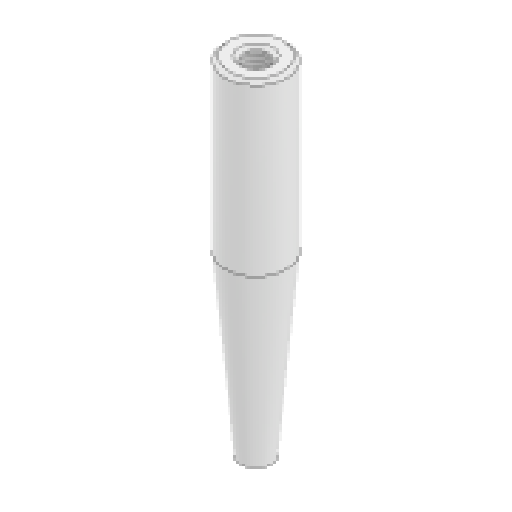
# Autodesk Inventor part: DLT-01-238B
Saved by Autodesk Inventor 2025.2 (Build 292293000, 293)
## iProperties
Company: Delta
Created: 2024-10-22
Part Number: DLT-01-238B
Material: Poliacetal WT
Document SubType Name: Modeling
Designer: Willian Pinheiro
Density: 1.4 g/cm^3
Appearance: Smooth - White
Project: DLT-01
Description: Dedo Pressor B
Mass: 13.0552 g
Surface Area: 40.3439 cm^2
Volume: 9.32516 cm^3
Acabamento: N/A
Dimensões: Ø10 x 45 mm
Total: 1
Author: Willian Pinheiro
Revision Number: 00
Autodesk Inventor part; units mm, degrees
ref_plane "YZ Plane" through (0, 0, 0) normal (1, 0, 0) x (0, 1, 0)
ref_plane "XZ Plane" through (0, 0, 0) normal (0, 1, 0) x (-1, 0, 0)
ref_plane "XY Plane" through (0, 0, 0) normal (0, 0, 1) x (1, 0, 0)
sketch "Sketch1" plane through (0, 0, 0) normal (0, 1, 0) x (-1, 0, 0)
  line L0 (4.8, 0) -> (-0.8, 0) construction
  line L1 (0, -37.7337) -> (0, 68.9023) construction
  line L2 (4, 22.5) -> (0, 22.5)
  line L3 (0, 22.5) -> (0, -22.5)
  line L4 (0, -22.5) -> (4, -22.5)
  line L5 (4, -22.5) -> (4, 22.5)
  line L6 (4, 53.6686) -> (4, 38.3314)
  line L7 (1.9878, -22.5) -> (4, 0.5)
  point P0 (0, 0)
  point P1 (0, 22.5)
  point P2 (0, -22.5)
  dimension "d2" = 8
  dimension "d5" = 23
  dimension "d21" = 45
  dimension "d22" = 3.9755
  dimension "d23" = 5
  constraints: 12 end point, 2 collinear, 2 parallel, 2 point on line, 1 horizontal, 1 perpendicular, 1 other
  measures "d2" diameter of L5 L1
  measures "d5" vertical distance of L7.start L7.end
  measures "d21" distance between parallel lines of L4 L2
  measures "d22" diameter of L7.start L1
  measures "d23" angle of L5 L7
revolve "Revolution1" add sketch "Sketch1" angle 360 about axis through (0, 0, -10) along (0, 0, 1) contours L5 L7 L4 L3 L2
sketch "Sketch2" plane through (0, 0, 22.5) normal (0, 0, 1) x (1, 0, 0)
  circle A0 centre (0, 0) radius 4 projected
  constraints: 1 coincident
hole "Hole1" at (0, 0, 22.5) direction (0, 0, -1) diameter 3.242 depth 25 tip angle 118 thread size "M4x0.7" class "6H" standard "ISO Metric profile"
chamfer "Chamfer1" distance 0.5 angle 45 2 edges at (4, 0, 22.5) (0, 1.621, 22.5)
body "Solid1"
